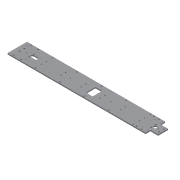
# Autodesk Inventor part: 1 Piece Support Plate
Saved by Autodesk Inventor 2011 (Build 150239000, 239)
## iProperties
Created: 2006-06-01
Part Number: 1 Piece Support Plate
Document SubType Name: Modeling
Designer: Jon
Density: 1 g/cm^3
Author: Jon
Autodesk Inventor part; units mm, degrees
ref_plane "YZ Plane" through (0, 0, 0) normal (1, 0, 0) x (0, 1, 0)
ref_plane "XZ Plane" through (0, 0, 0) normal (0, 1, 0) x (-1, 0, 0)
ref_plane "XY Plane" through (0, 0, 0) normal (0, 0, 1) x (1, 0, 0)
sketch "Sketch1" plane through (0, 0, 0) normal (0, 0, 1) x (1, 0, 0)
  line L0 (0, 0) -> (-757.71, 0)
  line L1 (-757.71, 0) -> (-757.71, 101.6)
  line L2 (-757.71, 101.6) -> (0, 101.6)
  line L3 (0, 101.6) -> (0, 0)
  dimension "d0" = 757.71
  dimension "d1" = 101.6
  constraints: 8 end point, 2 parallel, 1 horizontal, 1 perpendicular
  measures "d0" distance of L0.start L0.end
  measures "d1" distance of L2.end L0.start
extrude "Extrusion1" add sketch "Sketch1" along normal blind 6.35
sketch "Sketch2" plane through (0, 0, 6.35) normal (0, 0, 1) x (1, 0, 0)
  line L0 (-757.71, 0) -> (-757.71, 101.6) projected
  line L1 (-757.71, 101.6) -> (0, 101.6) projected
  line L2 (0, 0) -> (-757.71, 0) projected
  line L3 (0, 101.6) -> (0, 0) projected
  line L4 (-784.6272, 50.8) -> (38.5307, 50.8) construction
  line L5 (-757.71, 0) -> (-757.71, 101.6) projected
  line L6 (0, 0) -> (-757.71, 0) projected
  line L7 (0, 101.6) -> (0, 0) projected
  line L8 (-757.71, 101.6) -> (0, 101.6) projected
  circle A0 centre (-733.3565, 83.308) radius 2.15
  circle A1 centre (-683.3634, 82.4755) radius 2.15
  circle A2 centre (-684.4397, 17.8465) radius 2.15
  circle A3 centre (-734.4327, 18.679) radius 2.15
  point P0 (-732.31, 95.733)
  point P1 (-694.21, 95.733)
  point P2 (-694.21, 5.867)
  point P3 (-732.31, 5.867)
  point P4 (-618.162, 95.733)
  point P5 (-618.162, 5.867)
  point P6 (-618.162, 95.733)
  point P7 (-491.162, 95.733)
  point P8 (-491.162, 5.867)
  point P9 (-364.162, 95.733)
  point P10 (-364.162, 5.867)
  point P11 (-237.162, 95.733)
  point P12 (-237.162, 5.867)
  point P13 (-110.162, 95.733)
  point P14 (-110.162, 5.867)
  point P15 (-28.5772, 95.733)
  point P16 (-66.6772, 95.733)
  point P17 (-92.0772, 95.733)
  point P18 (-28.5772, 5.867)
  point P19 (-66.6772, 5.867)
  point P20 (-92.0772, 5.867)
  point P21 (-733.81, 63.246)
  point P22 (-733.81, 38.608)
  point P23 (-683.81, 63.246)
  point P24 (-683.81, 38.608)
  point P25 (-619.153, 63.246)
  point P26 (-619.153, 38.608)
  point P27 (-519.153, 63.246)
  point P28 (-519.153, 38.608)
  point P29 (-414.153, 63.246)
  point P30 (-414.153, 38.608)
  point P31 (-314.153, 63.246)
  point P32 (-314.153, 38.608)
  point P33 (-209.153, 63.246)
  point P34 (-209.153, 38.608)
  point P35 (-109.153, 63.246)
  point P36 (-109.153, 38.608)
  point P37 (-49.525, 63.246)
  point P38 (-49.525, 38.608)
  point P39 (-9.525, 38.608)
  point P40 (-9.525, 63.246)
  dimension "d4" = 50.8
  dimension "d5" = 38.1
  dimension "d6" = 25.4
  dimension "d7" = 5.867
  dimension "d8" = 5.867
  dimension "d9" = 76.048
  dimension "d10" = 127
  dimension "d11" = 127
  dimension "d12" = 127
  dimension "d13" = 127
  dimension "d15" = 38.1
  dimension "d16" = 25.4
  dimension "d24" = 50
  dimension "d25" = 23.9
  dimension "d26" = 24.638
  dimension "d27" = 38.608
  dimension "d28" = 100
  dimension "d30" = 100
  dimension "d31" = 105
  dimension "d32" = 105
  dimension "d33" = 100
  dimension "d34" = 18.0848
  dimension "d35" = 138.557
  dimension "d36" = 9.525
  dimension "d37" = 40
  constraints: 36 horizontal alignment, 20 vertical alignment, 5 coincident, 4 centre point, 2 end point, 1 perpendicular
  measures "d4" distance between parallel lines of L1 L4
  measures "d5" distance of point (-694.21, 95.733) point (-732.31, 95.733)
  measures "d6" distance from line of L0 point (-732.31, 95.733)
  measures "d7" vertical distance of L0.end point (-732.31, 95.733)
  measures "d8" distance from line of L2 point (-732.31, 5.867)
  measures "d9" distance of point (-618.162, 95.733) point (-694.21, 95.733)
  measures "d10" distance of point (-491.162, 95.733) point (-618.162, 95.733)
  measures "d11" distance of point (-364.162, 95.733) point (-491.162, 95.733)
  measures "d12" distance of point (-237.162, 95.733) point (-364.162, 95.733)
  measures "d13" distance of point (-110.162, 95.733) point (-237.162, 95.733)
  measures "d15" distance of point (-66.677, 95.733) point (-28.577, 95.733)
  measures "d16" distance of point (-92.077, 95.733) point (-66.677, 95.733)
  measures "d24" distance of point (-683.81, 38.608) point (-733.81, 38.608)
  measures "d25" distance from line of L0 point (-733.81, 38.608)
  measures "d26" distance of point (-683.81, 63.246) point (-683.81, 38.608)
  measures "d27" distance from line of L2 point (-733.81, 38.608)
  measures "d28" distance of point (-519.153, 38.608) point (-619.153, 38.608)
  measures "d30" distance of point (-314.153, 38.608) point (-414.153, 38.608)
  measures "d31" distance of point (-414.153, 38.608) point (-519.153, 38.608)
  measures "d32" distance of point (-209.153, 38.608) point (-314.153, 38.608)
  measures "d33" distance of point (-209.153, 38.608) point (-109.153, 38.608)
  measures "d34" distance of point (-92.077, 95.733) point (-110.162, 95.733)
  measures "d35" distance from line of point (-619.153, 38.608) L0
  measures "d36" distance from line of L3 point (-9.525, 38.608)
  measures "d37" distance of point (-49.525, 38.608) point (-9.525, 38.608)
hole "Hole1" at (-732.31, 95.733, 6.35) at (-694.21, 95.733, 6.35) at (-694.21, 5.867, 6.35) at (-732.31, 5.867, 6.35) at (-618.162, 95.733, 6.35) at (-618.162, 5.867, 6.35) at (-491.162, 95.733, 6.35) at (-491.162, 5.867, 6.35) at (-364.162, 95.733, 6.35) at (-364.162, 5.867, 6.35) at (-237.162, 95.733, 6.35) at (-237.162, 5.867, 6.35) at (-110.162, 95.733, 6.35) at (-110.162, 5.867, 6.35) at (-28.5772, 95.733, 6.35) at (-66.6772, 95.733, 6.35) at (-92.0772, 95.733, 6.35) at (-28.5772, 5.867, 6.35) at (-66.6772, 5.867, 6.35) at (-92.0772, 5.867, 6.35) direction (0, 0, -1) diameter 7.6 end through all
hole "Hole3" at (-619.153, 38.608, 6.35) at (-619.153, 63.246, 6.35) at (-519.153, 63.246, 6.35) at (-519.153, 38.608, 6.35) at (-414.153, 63.246, 6.35) at (-414.153, 38.608, 6.35) at (-314.153, 63.246, 6.35) at (-314.153, 38.608, 6.35) at (-109.153, 63.246, 6.35) at (-109.153, 38.608, 6.35) at (-209.153, 38.608, 6.35) at (-209.153, 63.246, 6.35) direction (0, 0, -1) diameter 6.7 end through all
hole "Hole4" at (-733.81, 63.246, 6.35) at (-733.81, 38.608, 6.35) at (-683.81, 63.246, 6.35) at (-683.81, 38.608, 6.35) at (-49.525, 63.246, 6.35) at (-49.525, 38.608, 6.35) at (-9.525, 38.608, 6.35) at (-9.525, 63.246, 6.35) direction (0, 0, -1) diameter 7.9375 end through all
sketch "Sketch3" plane through (0, 0, 6.35) normal (0, 0, 1) x (1, 0, 0)
  line L0 (-757.71, 0) -> (-757.71, 101.6) projected
  line L1 (-757.71, 101.6) -> (0, 101.6) projected
  line L2 (0, 0) -> (-757.71, 0) projected
  line L3 (0, 101.6) -> (0, 0) projected
  line L4 (-768.3938, 50.8) -> (17.8568, 50.8) construction
  circle A0 centre (-364.162, 95.733) radius 3.8 construction
  circle A1 centre (-364.162, 5.867) radius 3.8 construction
  line L5 (-678.81, 101.6) -> (-678.81, 0) construction
  line L6 (-658.81, 101.6) -> (-658.81, 0) construction
  line L7 (-678.81, 58.8) -> (-658.81, 58.8)
  line L8 (-658.81, 42.8) -> (-678.81, 42.8)
  arc A2 (-678.81, 58.8) -> (-678.81, 42.8) centre (-678.81, 50.8) ccw
  arc A3 (-658.81, 42.8) -> (-658.81, 58.8) centre (-658.81, 50.8) ccw
  line L9 (-358.637, 61.5353) -> (-358.637, 20.4895) construction
  line L10 (-374.137, 75.8) -> (-343.137, 75.8)
  line L11 (-341.137, 73.8) -> (-341.137, 27.8)
  line L12 (-343.137, 25.8) -> (-374.137, 25.8)
  line L13 (-376.137, 27.8) -> (-376.137, 73.8)
  arc A4 (-374.137, 75.8) -> (-376.137, 73.8) centre (-374.137, 73.8) ccw
  arc A5 (-341.137, 73.8) -> (-343.137, 75.8) centre (-343.137, 73.8) ccw
  arc A6 (-343.137, 25.8) -> (-341.137, 27.8) centre (-343.137, 27.8) ccw
  arc A7 (-376.137, 27.8) -> (-374.137, 25.8) centre (-374.137, 27.8) ccw
  point P0 (-376.137, 75.8)
  point P1 (-341.137, 75.8)
  point P2 (-376.137, 25.8)
  dimension "d59" = 50.8
  dimension "d65" = 78.9
  dimension "d66" = 20
  dimension "d67" = 8
  dimension "d68" = 16
  dimension "d110" = 35
  dimension "d111" = 50
  dimension "d112" = 17.5
  dimension "d113" = 25
  dimension "d115" = 2
  dimension "d118" = 399.073
  constraints: 20 end point, 12 point on circle, 12 point on line, 12 tangent, 6 centre point, 5 perpendicular, 4 parallel, 3 equal radius, 1 horizontal
  measures "d59" distance from line of L4 L0.end
  measures "d65" distance between parallel lines of L5 L0
  measures "d66" distance between parallel lines of L6 L5
  measures "d67" distance between parallel lines of L7 L4
  measures "d68" distance between parallel lines of L8 L7
  measures "d110" distance of point (-376.137, 75.8) point (-341.137, 75.8)
  measures "d111" distance of point (-376.137, 25.8) point (-376.137, 75.8)
  measures "d112" distance between parallel lines of L13 L9
  measures "d113" distance between parallel lines of L12 L4
  measures "d115" radius of A4
  measures "d118" distance between parallel lines of L9 L0
sketch "Sketch5" plane through (0, 0, 6.35) normal (0, 0, 1) x (1, 0, 0)
  line L0 (-58.4858, 50.8) -> (0.3179, 50.8) construction
  line L1 (-757.71, 101.6) -> (0, 101.6) construction
  line L2 (0, 101.6) -> (0, 0) construction
  point P0 (-40.919, 50.8)
  dimension "d84" = 50.8
  dimension "d86" = 40.919
  constraints: 2 end point, 1 horizontal, 1 point on line
  measures "d84" distance between parallel lines of L0 L1
  measures "d86" distance from line of point (-40.919, 50.8) L2
hole "Hole6" at (-40.919, 50.8, 6.35) direction (0, 0, -1) diameter 17.78 end through all
sketch "Sketch6" plane through (0, 0, 6.35) normal (0, 0, 1) x (1, 0, 0)
  circle A0 centre (-40.919, 50.8) radius 8.89 construction
  line L0 (0, 101.6) -> (0, 0) construction
  line L1 (-40.919, 50.8) -> (0, 50.8) construction
  point P0 (-23.825, 50.8)
  dimension "d95" = 23.825
  constraints: 2 end point, 1 midpoint, 1 point on line
  measures "d95" distance from line of point (-23.825, 50.8) L0
hole "Hole7" at (-23.825, 50.8, 6.35) direction (0, 0, -1) diameter 3 end through all
extrude "Extrusion3" cut sketch "Sketch3" against normal through all contours L7 A3 L8 A2 | L10 A5 L11 A6 L12 A7 L13 A4
sketch "Sketch7" plane through (0, 0, 6.35) normal (0, 0, 1) x (1, 0, 0)
  arc A0 (-678.81, 58.8) -> (-678.81, 42.8) centre (-678.81, 50.8) ccw projected
  line L0 (-678.81, 58.8) -> (-658.81, 58.8) projected
  arc A1 (-658.81, 42.8) -> (-658.81, 58.8) centre (-658.81, 50.8) ccw projected
  line L1 (-658.81, 42.8) -> (-678.81, 42.8) projected
  line L2 (-376.137, 27.8) -> (-376.137, 73.8) projected
  arc A2 (-374.137, 75.8) -> (-376.137, 73.8) centre (-374.137, 73.8) ccw projected
  line L3 (-374.137, 75.8) -> (-343.137, 75.8) projected
  arc A3 (-341.137, 73.8) -> (-343.137, 75.8) centre (-343.137, 73.8) ccw projected
  line L4 (-341.137, 73.8) -> (-341.137, 27.8) projected
  arc A4 (-343.137, 25.8) -> (-341.137, 27.8) centre (-343.137, 27.8) ccw projected
  line L5 (-343.137, 25.8) -> (-374.137, 25.8) projected
  arc A5 (-376.137, 27.8) -> (-374.137, 25.8) centre (-374.137, 27.8) ccw projected
  circle A6 centre (-23.825, 50.8) radius 1.5 projected
  circle A7 centre (-40.919, 50.8) radius 8.89 projected
  circle A8 centre (-9.525, 38.608) radius 3.9688 projected
  circle A9 centre (-49.525, 63.246) radius 3.9688 projected
  circle A10 centre (-683.81, 63.246) radius 3.9688 projected
  circle A11 centre (-733.81, 63.246) radius 3.9688 projected
  circle A12 centre (-733.81, 38.608) radius 3.9688 projected
  circle A13 centre (-683.81, 38.608) radius 3.9688 projected
  circle A14 centre (-49.525, 38.608) radius 3.9688 projected
  circle A15 centre (-9.525, 63.246) radius 3.9688 projected
  circle A16 centre (-209.153, 38.608) radius 3.35 projected
  circle A17 centre (-109.153, 63.246) radius 3.35 projected
  circle A18 centre (-314.153, 63.246) radius 3.35 projected
  circle A19 centre (-414.153, 63.246) radius 3.35 projected
  circle A20 centre (-519.153, 63.246) radius 3.35 projected
  circle A21 centre (-619.153, 38.608) radius 3.35 projected
  circle A22 centre (-619.153, 63.246) radius 3.35 projected
  circle A23 centre (-519.153, 38.608) radius 3.35 projected
  circle A24 centre (-414.153, 38.608) radius 3.35 projected
  circle A25 centre (-314.153, 38.608) radius 3.35 projected
  circle A26 centre (-109.153, 38.608) radius 3.35 projected
  circle A27 centre (-209.153, 63.246) radius 3.35 projected
  circle A28 centre (-66.6772, 5.867) radius 3.8 projected
  circle A29 centre (-92.0772, 95.733) radius 3.8 projected
  circle A30 centre (-28.5772, 95.733) radius 3.8 projected
  circle A31 centre (-110.162, 95.733) radius 3.8 projected
  circle A32 centre (-237.162, 95.733) radius 3.8 projected
  circle A33 centre (-364.162, 95.733) radius 3.8 projected
  circle A34 centre (-491.162, 95.733) radius 3.8 projected
  circle A35 centre (-618.162, 95.733) radius 3.8 projected
  circle A36 centre (-694.21, 5.867) radius 3.8 projected
  circle A37 centre (-732.31, 95.733) radius 3.8 projected
  circle A38 centre (-694.21, 95.733) radius 3.8 projected
  circle A39 centre (-732.31, 5.867) radius 3.8 projected
  circle A40 centre (-618.162, 5.867) radius 3.8 projected
  circle A41 centre (-491.162, 5.867) radius 3.8 projected
  circle A42 centre (-364.162, 5.867) radius 3.8 projected
  circle A43 centre (-237.162, 5.867) radius 3.8 projected
  circle A44 centre (-110.162, 5.867) radius 3.8 projected
  circle A45 centre (-66.6772, 95.733) radius 3.8 projected
  circle A46 centre (-28.5772, 5.867) radius 3.8 projected
  circle A47 centre (-92.0772, 5.867) radius 3.8 projected
  line L6 (-757.71, 0) -> (-757.71, 101.6) projected
  line L7 (0, 0) -> (-757.71, 0) projected
  line L8 (0, 101.6) -> (0, 0) projected
  line L9 (-757.71, 101.6) -> (0, 101.6) projected
  point P0 (-708.71, 50.8)
  point P1 (-480.71, 50.8)
  point P2 (-268.919, 50.8)
  point P3 (-24, 50.8)
  dimension "d119" = 49
  dimension "d120" = 228
  dimension "d121" = 228
  dimension "d122" = 24
  constraints: 4 horizontal alignment
  measures "d119" distance from line of point (-708.71, 50.8) L6
  measures "d120" distance of point (-480.71, 50.8) point (-708.71, 50.8)
  measures "d121" distance of point (-268.919, 50.8) A7.centre
  measures "d122" distance from line of L8 point (-24, 50.8)
hole "Hole8" at (-708.71, 50.8, 6.35) at (-480.71, 50.8, 6.35) at (-268.919, 50.8, 6.35) at (-24, 50.8, 6.35) direction (0, 0, -1) diameter 5.1 end through all
sketch "Sketch8" plane through (0, 0, 6.35) normal (0, 0, 1) x (1, 0, 0)
  circle A0 centre (-268.919, 50.8) radius 2.55 projected
  circle A1 centre (-708.71, 50.8) radius 2.55 projected
  circle A2 centre (-480.71, 50.8) radius 2.55 projected
  circle A3 centre (-24, 50.8) radius 2.55 projected
  arc A4 (-678.81, 58.8) -> (-678.81, 42.8) centre (-678.81, 50.8) ccw projected
  line L0 (-678.81, 58.8) -> (-658.81, 58.8) projected
  arc A5 (-658.81, 42.8) -> (-658.81, 58.8) centre (-658.81, 50.8) ccw projected
  line L1 (-658.81, 42.8) -> (-678.81, 42.8) projected
  line L2 (-376.137, 27.8) -> (-376.137, 73.8) projected
  arc A6 (-374.137, 75.8) -> (-376.137, 73.8) centre (-374.137, 73.8) ccw projected
  line L3 (-374.137, 75.8) -> (-343.137, 75.8) projected
  arc A7 (-341.137, 73.8) -> (-343.137, 75.8) centre (-343.137, 73.8) ccw projected
  line L4 (-341.137, 73.8) -> (-341.137, 27.8) projected
  arc A8 (-343.137, 25.8) -> (-341.137, 27.8) centre (-343.137, 27.8) ccw projected
  line L5 (-343.137, 25.8) -> (-374.137, 25.8) projected
  arc A9 (-376.137, 27.8) -> (-374.137, 25.8) centre (-374.137, 27.8) ccw projected
  circle A10 centre (-40.919, 50.8) radius 8.89 projected
  circle A11 centre (-9.525, 38.608) radius 3.9688 projected
  circle A12 centre (-49.525, 63.246) radius 3.9688 projected
  circle A13 centre (-683.81, 63.246) radius 3.9688 projected
  circle A14 centre (-733.81, 63.246) radius 3.9688 projected
  circle A15 centre (-733.81, 38.608) radius 3.9688 projected
  circle A16 centre (-683.81, 38.608) radius 3.9688 projected
  circle A17 centre (-49.525, 38.608) radius 3.9688 projected
  circle A18 centre (-9.525, 63.246) radius 3.9688 projected
  circle A19 centre (-209.153, 38.608) radius 3.35 projected
  circle A20 centre (-109.153, 63.246) radius 3.35 projected
  circle A21 centre (-314.153, 63.246) radius 3.35 projected
  circle A22 centre (-414.153, 63.246) radius 3.35 projected
  circle A23 centre (-519.153, 63.246) radius 3.35 projected
  circle A24 centre (-619.153, 38.608) radius 3.35 projected
  circle A25 centre (-619.153, 63.246) radius 3.35 projected
  circle A26 centre (-519.153, 38.608) radius 3.35 projected
  circle A27 centre (-414.153, 38.608) radius 3.35 projected
  circle A28 centre (-314.153, 38.608) radius 3.35 projected
  circle A29 centre (-109.153, 38.608) radius 3.35 projected
  circle A30 centre (-209.153, 63.246) radius 3.35 projected
  circle A31 centre (-66.6772, 5.867) radius 3.8 projected
  circle A32 centre (-92.0772, 95.733) radius 3.8 projected
  circle A33 centre (-28.5772, 95.733) radius 3.8 projected
  circle A34 centre (-110.162, 95.733) radius 3.8 projected
  circle A35 centre (-237.162, 95.733) radius 3.8 projected
  circle A36 centre (-364.162, 95.733) radius 3.8 projected
  circle A37 centre (-491.162, 95.733) radius 3.8 projected
  circle A38 centre (-618.162, 95.733) radius 3.8 projected
  circle A39 centre (-694.21, 5.867) radius 3.8 projected
  circle A40 centre (-732.31, 95.733) radius 3.8 projected
  circle A41 centre (-694.21, 95.733) radius 3.8 projected
  circle A42 centre (-732.31, 5.867) radius 3.8 projected
  circle A43 centre (-618.162, 5.867) radius 3.8 projected
  circle A44 centre (-491.162, 5.867) radius 3.8 projected
  circle A45 centre (-364.162, 5.867) radius 3.8 projected
  circle A46 centre (-237.162, 5.867) radius 3.8 projected
  circle A47 centre (-110.162, 5.867) radius 3.8 projected
  circle A48 centre (-66.6772, 95.733) radius 3.8 projected
  circle A49 centre (-28.5772, 5.867) radius 3.8 projected
  circle A50 centre (-92.0772, 5.867) radius 3.8 projected
  line L6 (-757.71, 0) -> (-757.71, 101.6) projected
  line L7 (0, 0) -> (-757.71, 0) projected
  line L8 (0, 101.6) -> (0, 0) projected
  line L9 (-757.71, 101.6) -> (0, 101.6) projected
  line L10 (0, 101.6) -> (-40, 101.6)
  line L11 (-40, 101.6) -> (-40, 76.6)
  line L12 (-40, 76.6) -> (0, 76.6)
  line L13 (0, 76.6) -> (0, 101.6)
  line L14 (0, 0) -> (-40, 0)
  line L15 (-40, 0) -> (-40, 25)
  line L16 (-40, 25) -> (0, 25)
  line L17 (0, 25) -> (0, 0)
  dimension "d130" = 40
  dimension "d131" = 25
  dimension "d132" = 25
  constraints: 16 end point, 4 parallel, 2 horizontal, 2 perpendicular, 1 collinear
  measures "d130" distance between parallel lines of L13 L11
  measures "d131" distance between parallel lines of L10 L12
  measures "d132" distance between parallel lines of L7 L16
extrude "Extrusion4" cut sketch "Sketch8" against normal through all contours L15 L16 L8 L7 | L9 L8 L12 L11
sketch "Sketch11" plane through (0, 0, 6.35) normal (0, 0, 1) x (1, 0, 0)
  line L0 (-40, 0) -> (-40, 25) projected
  line L1 (-40, 76.6) -> (-40, 101.6) projected
  line L2 (-757.71, 101.6) -> (-40, 101.6) projected
  line L3 (-757.71, 0) -> (-757.71, 101.6) projected
  line L4 (-40, 0) -> (-757.71, 0) projected
  point P0 (0, 0)
  point P1 (-733.71, 81.8)
  point P2 (-683.71, 81.8)
  point P3 (-683.71, 19.8)
  point P4 (-733.71, 19.8)
  point P5 (-45.71, 82.8)
  point P6 (-72.71, 82.8)
  point P7 (-72.71, 18.8)
  point P8 (-45.71, 18.8)
  dimension "d149" = 19.8
  dimension "d150" = 19.8
  dimension "d151" = 19.8
  dimension "d152" = 19.8
  dimension "d153" = 24
  dimension "d154" = 24
  dimension "d155" = 50
  dimension "d156" = 50
  dimension "d157" = 18.8
  dimension "d158" = 18.8
  dimension "d159" = 18.8
  dimension "d160" = 18.8
  dimension "d161" = 5.71
  dimension "d162" = 5.71
  dimension "d172" = 27
  dimension "d173" = 27
  measures "d149" distance from line of L2 point (-733.71, 81.8)
  measures "d150" distance from line of L2 point (-683.71, 81.8)
  measures "d151" distance from line of L4 point (-683.71, 19.8)
  measures "d152" distance from line of point (-733.71, 19.8) L4
  measures "d153" distance from line of point (-733.71, 19.8) L3
  measures "d154" distance from line of point (-733.71, 81.8) L3
  measures "d155" distance of point (-733.71, 81.8) point (-683.71, 81.8)
  measures "d156" distance of point (-733.71, 19.8) point (-683.71, 19.8)
  measures "d157" distance from line of point (-72.71, 82.8) L2
  measures "d158" distance from line of L2 point (-45.71, 82.8)
  measures "d159" distance from line of L4 point (-72.71, 18.8)
  measures "d160" distance from line of point (-45.71, 18.8) L4
  measures "d161" distance from line of point (-45.71, 18.8) L0
  measures "d162" distance from line of point (-45.71, 82.8) L1
  measures "d172" distance of point (-72.71, 82.8) point (-45.71, 82.8)
  measures "d173" distance of point (-72.71, 18.8) point (-45.71, 18.8)
hole "Hole11" at (-733.71, 81.8, 6.35) at (-683.71, 81.8, 6.35) at (-683.71, 19.8, 6.35) at (-733.71, 19.8, 6.35) at (-45.71, 82.8, 6.35) at (-72.71, 82.8, 6.35) at (-72.71, 18.8, 6.35) at (-45.71, 18.8, 6.35) direction (0, 0, -1) diameter 4.3 end through all
equation "\"d8\" = d7"
equation "\"d11\" = d10"
equation "\"d12\" = d10"
equation "\"d13\" = d10"
equation "\"d132\" = d131"
equation "\"d150\" = d149"
equation "\"d151\" = d149"
equation "\"d152\" = d149"
equation "\"d154\" = d153"
equation "\"d156\" = d155"
equation "\"d158\" = d157"
equation "\"d159\" = d157"
equation "\"d160\" = d157"
body "Solid1"
